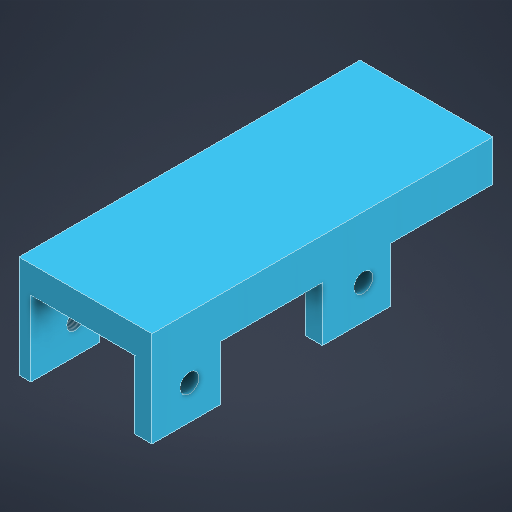
# Autodesk Inventor part: Befestigung Bremssattel
Saved by Autodesk Inventor 2026.2 (Build 302298010, 298A)
## iProperties
Created: 2026-04-15
Part Number: Befestigung Bremssattel
Material: Generisch
Document SubType Name: Modeling
Designer: pparr
Density: 1 g/cm^3
Appearance: Türkis
Author: pparr
Autodesk Inventor part; units mm, degrees
ref_plane "YZ Plane" through (0, 0, 0) normal (1, 0, 0) x (0, 1, 0)
ref_plane "XZ Plane" through (0, 0, 0) normal (0, 1, 0) x (-1, 0, 0)
ref_plane "XY Plane" through (0, 0, 0) normal (0, 0, 1) x (1, 0, 0)
sketch "Skizze1" plane through (0, 0, 0) normal (0, 1, 0) x (-1, 0, 0)
  line L0 (0, 0) -> (0, 8)
  line L1 (0, 8) -> (2, 8)
  line L2 (2, 8) -> (2, 4)
  line L3 (2, 4) -> (39, 4)
  line L4 (39, 4) -> (39, 0)
  line L5 (0, 0) -> (13.2064, 0)
  line L6 (0, 0) -> (0, -8)
  line L7 (0, -8) -> (2, -8)
  line L8 (2, -8) -> (2, -4)
  line L9 (2, -4) -> (39, -4)
  line L10 (39, -4) -> (39, 0)
  dimension "d1" = 8
  dimension "d2" = 2
  dimension "d3" = 4
  dimension "d4" = 37
  constraints: 22 end point, 4 symmetric about line, 3 perpendicular, 2 vertical, 1 horizontal
  measures "d1" distance of L0.start L0.end
  measures "d2" distance of L0.end L1.end
  measures "d3" distance of L1.end L2.end
  measures "d4" distance of L2.end L3.end
extrude "Extrusion1" add sketch "Skizze1" along normal mid plane 100
sketch "Skizze5" plane through (-39, -50, 4) normal (0, 0, 1) x (1, 0, 0)
  line L0 (0, 0) -> (0, 100) projected
  line L1 (0, 0) -> (3.5, 0)
  line L2 (3.5, 0) -> (3.5, 20)
  line L3 (3.5, 20) -> (0, 20)
  line L4 (0, 20) -> (0, 0)
  point P0 (39, 50)
  point P1 (0, 20.0912)
  dimension "d22" = 3.5
  dimension "d23" = 20
  constraints: 8 end point, 2 parallel, 1 horizontal, 1 perpendicular
  measures "d22" distance of L3.end L2.end
  measures "d23" distance of L2.end L1.end
extrude "Extrusion3" add sketch "Skizze5" along normal blind 20 and the other way blind 30
sketch "Skizze6" plane through (-39, 50, 4) normal (0, 0, 1) x (1, 0, 0)
  line L0 (0, -80) -> (0, 0) projected
  line L1 (0, 0) -> (3.5, 0)
  line L2 (3.5, 0) -> (3.5, -20)
  line L3 (3.5, -20) -> (0, -20)
  line L4 (0, -20) -> (0, 0)
  point P0 (39, -50)
  point P1 (0, -19.9088)
  point P2 (0, -20)
  dimension "d26" = 20
  dimension "d32" = 3.5
  constraints: 8 end point, 2 parallel, 1 horizontal, 1 perpendicular
  measures "d26" distance of L1.end L2.end
  measures "d32" distance between parallel lines of L0 L2
extrude "Extrusion4" add sketch "Skizze6" along normal blind 20 and the other way blind 30
sketch "Esquisse11" plane through (-35.5, 30, -4) normal (1, 0, 0) x (0, 0, -1)
  line L0 (22, 20) -> (0, 20) projected
  line L1 (22, 20) -> (22, 0) projected
  line L2 (22, -60) -> (22, -80) projected
  point P0 (-4, -30)
  point P1 (13, 7)
  point P2 (13, -67)
  dimension "d57" = 13
  dimension "d58" = 74
  dimension "d59" = 9
  dimension "d60" = 9
  measures "d57" distance from line of point (13, 7) L0
  measures "d58" distance of point (13, -67) point (13, 7)
  measures "d59" distance from line of L1 point (13, 7)
  measures "d60" distance from line of L2 point (13, -67)
hole "Perçage3" at (-35.5, 37, -17) at (-35.5, -37, -17) direction (-1, 0, 0) diameter 4.917 end through all thread size "M6x1" class "6H" standard "ISO Metric profile"
sketch "Esquisse21" plane through (-35.5, -50, 4) normal (1, 0, 0) x (0, 0, -1)
  line L0 (0, 100) -> (0, 80) projected
  line L1 (0, 20) -> (0, 80) projected
  line L2 (0, 20) -> (0, 0) projected
  line L3 (0, 100) -> (0, 0) projected
  line L4 (-36.3372, 0) -> (0, 0)
  line L5 (0, 0) -> (0, 115.7943)
  line L6 (0, 115.7943) -> (-36.3372, 115.7943)
  line L7 (-36.3372, 115.7943) -> (-36.3372, 0)
  point P0 (4, 50)
  point P1 (0, 20)
  constraints: 8 end point, 2 parallel, 1 horizontal, 1 perpendicular
extrude "Extrusion15" cut sketch "Esquisse21" along normal mid plane 9999
sketch "Esquisse22" plane through (-2, -50, -4) normal (0, 0, -1) x (-1, 0, 0)
  line L0 (37, 15.4585) -> (37, 10.5415) projected
  line L1 (33.5, 10.5415) -> (33.5, 15.4585) projected
  line L2 (-2, 0) -> (3, 0)
  line L3 (3, 0) -> (3, 20)
  line L4 (3, 20) -> (-2, 20)
  line L5 (-2, 20) -> (-2, 0)
  line L6 (33.5, 0) -> (0, 0) projected
  line L7 (-2, 0) -> (-2, 100) projected
  point P0 (-2, 50)
  point P1 (0.5, 0)
  dimension "d92" = 5
  dimension "d93" = 0
  dimension "d94" = 0
  constraints: 8 end point, 2 parallel, 1 horizontal, 1 midpoint, 1 perpendicular
  measures "d92" distance of L3.end L4.end
  measures "d93" distance from line of L6 point (0.5, 0)
  measures "d94" distance between parallel lines of L7 L5
extrude "Extrusion16" add sketch "Esquisse22" along normal blind 20
sketch "Esquisse23" plane through (-5, -50, -4) normal (-1, 0, 0) x (0, 0, 1)
  line L0 (0, 20) -> (-20, 20) projected
  line L1 (-20, 0) -> (-20, 20) projected
  point P0 (4, 50)
  point P1 (-10, 11)
  dimension "d104" = 9
  dimension "d105" = 10
  measures "d104" distance from line of L0 point (-10, 11)
  measures "d105" distance from line of L1 point (-10, 11)
hole "Perçage5" at (-5, -39, -14) direction (1, 0, 0) diameter 5.5 end through all clearance for "Vis à tête plate fraisée ISO 2009/7046" size "M5" standard "ISO"
sketch "Esquisse24" plane through (-35.5, -30, -4) normal (0, 0, -1) x (-1, 0, 0)
  line L0 (-35.5, 0) -> (-35.5, 80) projected
  line L1 (-35.5, 50) -> (-30.5, 50)
  line L2 (-30.5, 50) -> (-30.5, 30)
  line L3 (-30.5, 30) -> (-35.5, 30)
  line L4 (-35.5, 30) -> (-35.5, 50)
  line L5 (-30.5, 0) -> (-35.5, 0) projected
  point P0 (-35.5, 30)
  dimension "d106" = 5
  dimension "d107" = 20
  dimension "d108" = 30
  constraints: 8 end point, 2 parallel, 1 horizontal, 1 perpendicular, 1 point on line
  measures "d106" distance of L2.end L3.end
  measures "d107" distance of L1.end L2.end
  measures "d108" distance between parallel lines of L5 L3
extrude "Extrusion17" add sketch "Esquisse24" along normal blind 20
sketch "Esquisse25" plane through (-5, 0, -4) normal (-1, 0, 0) x (0, 0, 1)
  line L0 (-20, 0) -> (-20, 20) projected
  line L1 (0, 20) -> (-20, 20) projected
  point P0 (4, 0)
  point P1 (-10, 12)
  dimension "d118" = 10
  dimension "d119" = 8
  measures "d118" distance from line of L0 point (-10, 12)
  measures "d119" distance from line of L1 point (-10, 12)
hole "Perçage6" at (-5, 12, -14) direction (1, 0, 0) diameter 5.5 end through all clearance for "Vis à tête plate fraisée ISO 2009/7046" size "M5" standard "ISO"
